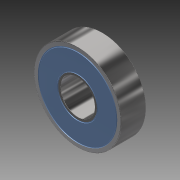
# Autodesk Inventor part: SHU63_22RS
Saved by Autodesk Inventor 2014 (Build 180170000, 170)
## iProperties
Category: Miscellaneous
Company: Autodesk Inc.
Created: 2013-12-28
Part Number: SHU63_22RS
Material: Stainless Steel, 440C
Document SubType Name: Modeling
Designer: Autodesk Inc.
Density: 7.75 g/cm^3
Appearance: Steel - Polished
Catalog Web Link: http://www.shusterbearings.com/shopexd.asp?id=98
Vendor: Shuster
Author: Autodesk Inc.
Autodesk Inventor part; units mm, degrees
ref_plane "YZ Plane" through (0, 0, 0) normal (1, 0, 0) x (0, 1, 0)
ref_plane "XZ Plane" through (0, 0, 0) normal (0, 1, 0) x (-1, 0, 0)
sketch "Sketch1" plane through (0, 0, 0) normal (0, 1, 0) x (-1, 0, 0)
  circle A0 centre (0, 0) radius 11
  circle A1 centre (0, 0) radius 28
  dimension "d0" = 22
  dimension "d1" = 56
  constraints: 2 centre point, 2 coincident
  measures "d0" diameter of A0
  measures "d1" diameter of A1
extrude "Extrusion1" add sketch "Sketch1" against normal blind 16
fillet "Fillet1" radius 0.3 4 edges at (28, 0, 0) (28, -16, 0) (11, 0, 0) (11, -16, 0)
sketch "Sketch2" plane through (0, 0, 0) normal (1, 0, 0) x (0, 1, 0)
  line L0 (-16, -27.7) -> (-16, 27.7) projected
  line L1 (-0.3, 28) -> (-15.7, 28) projected
  circle A0 centre (-16, 25.1814) radius 0.3168
  circle A1 centre (-16, 12.7277) radius 0.3168
  line L2 (-18.3802, 0) -> (3.0634, 0) projected
  point P0 (0, 0)
  constraints: 2 centre point, 2 point on line, 1 equal radius
revolve "Revolution1" cut sketch "Sketch2" angle 360 about axis through (0, -10, 0) along (0, 1, 0)
ref_plane "Work Plane1" through (0, -8, 0) normal (0, 1, 0) x (1, 0, 0)
mirror "Mirror1" about plane through (0, -8, 0) normal (0, 1, 0) of "Revolution1"
body "Solid1"
